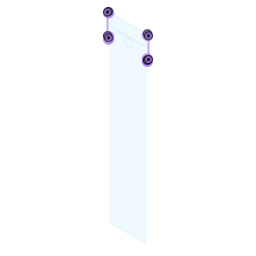
final project_ duck lamp (Autodesk Fusion 360 design; units mm, degrees)
Autodesk Fusion 360 part; units mm, degrees
note: some values were not read from the file. Set by a fixed rule: which sketch regions a step uses.
sketch "Sketch1" plane through (0, 0, 0) normal (0, 1, 0) x (1, 0, 0) in component "back piece"
  line L0 (0, 0) -> (80, 0)
  line L1 (80, 0) -> (80, -347.5)
  line L2 (80, -400) -> (0, -400)
  line L3 (0, -347.5) -> (0, 0)
  line L4 (9, 0) -> (11, 0)
  line L5 (75, -375) -> (5, -375)
  line L6 (5, -375) -> (5, -372)
  line L7 (5, -372) -> (75, -372)
  line L8 (75, -372) -> (75, -375)
  circle A0 centre (40, -363.2398) radius 8.7602
  line L9 (44.9524, -352.3526) -> (35, -352.3526)
  line L10 (35, -352.3526) -> (35, 0)
  line L11 (35, 0) -> (44.9524, 0)
  line L12 (44.9524, 0) -> (44.9524, -352.3526)
  line L13 (0, 0) -> (3, 0)
  line L14 (3, 0) -> (3, -3)
  line L15 (3, -3) -> (0, -3)
  line L16 (80, 0) -> (77, 0)
  line L17 (77, 0) -> (77, -3)
  line L18 (77, -3) -> (80, -3)
  line L19 (80, -3) -> (80, 0)
  line L20 (85, -352.5) -> (85, -397.5)
  line L21 (82.5, -400) -> (-2.5, -400)
  line L22 (-5, -397.5) -> (-5, -352.5)
  line L23 (-2.4999, -350) -> (-2.5, -350)
  line L24 (82.4999, -350) -> (82.5001, -350)
  arc A1 (-2.5, -350) -> (0, -347.5) centre (-2.5, -347.5) ccw
  arc A2 (80, -347.5) -> (82.4999, -350) centre (82.5, -347.5) ccw
  arc A3 (-2.4999, -350) -> (-5, -352.5) centre (-2.5, -352.5) ccw
  arc A4 (85, -352.5) -> (82.5001, -350) centre (82.5, -352.5) ccw
  arc A5 (-5, -397.5) -> (-2.5, -400) centre (-2.5, -397.5) ccw
  arc A6 (82.5, -400) -> (85, -397.5) centre (82.5, -397.5) ccw
  dimension "d5" = 400
  dimension "d6" = 80
  dimension "d98" = 3
  dimension "d99" = 70
  dimension "d115" = 3
  dimension "d116" = 3
  dimension "d117" = 3
  dimension "d118" = 3
  dimension "d121" = 2.5
  dimension "d122" = 2.5
  dimension "d123" = 2.5
  dimension "d124" = 2.5
  dimension "d125" = 2.5
  dimension "d126" = 2.5
  constraint horizontal L0
  constraint vertical L1
  constraint horizontal L2
  constraint vertical L3
  constraint coincident L0.start L3.end
  constraint horizontal L4
  constraint coincident L0 L4.start
  constraint horizontal L5
  constraint vertical L6
  constraint horizontal L7
  constraint vertical L8
  constraint tangent L7 A0
  constraint horizontal L9
  constraint vertical L10
  constraint horizontal L11
  constraint vertical L12
  constraint coincident L0 L10.end
  constraint horizontal L13
  constraint vertical L14
  constraint horizontal L15
  constraint horizontal L16
  constraint vertical L17
  constraint horizontal L18
  constraint vertical L19
  constraint vertical L20
  constraint horizontal L21
  constraint vertical L22
  constraint tangent L3 A1
  constraint tangent L1 A2
  constraint tangent L22 A3
  constraint tangent L20 A4
  constraint tangent L24 A4
  constraint tangent L22 A5
  constraint tangent L21 A5
  constraint tangent L21 A6
  constraint tangent L20 A6
  measures "d5" distance of L0 L2
  measures "d6" distance of L1 L3
  measures "d98" distance of L5 L7
  measures "d99" distance of L6 L8
  measures "d115" distance of L3 L14
  measures "d116" distance of L0 L15
  measures "d117" distance of L0 L18
  measures "d118" distance of L1 L17
  measures "d121" radius of A1
  measures "d122" radius of A2
  measures "d123" radius of A3
  measures "d124" radius of A4
  measures "d125" radius of A5
  measures "d126" radius of A6
sketch "Sketch1 (2)" plane through (0, 0, 0) normal (0, 0, 1) x (1, 0, 0) in component "bottom base"
  line L0 (0, 0) -> (200, 0)
  line L1 (200, 0) -> (200, 106)
  line L2 (200, 106) -> (0, 106)
  line L3 (0, 106) -> (0, 0)
  circle A0 centre (158.3517, 50) radius 35.4262
  circle A1 centre (78.412, 50) radius 35.3232
  line L4 (28.714, 90) -> (25.714, 90)
  line L5 (25.714, 90) -> (25.714, 16)
  line L6 (25.714, 16) -> (28.714, 16)
  line L7 (28.714, 16) -> (28.714, 90)
  dimension "d8" = 200
  dimension "d11" = 106
  dimension "d110" = 3
  dimension "d111" = 74
  dimension "d112" = 16
  dimension "d113" = 10
  dimension "d114" = 25.714
  constraint horizontal L0
  constraint vertical L1
  constraint horizontal L2
  constraint vertical L3
  constraint coincident L0.start L3.end
  constraint horizontal L4
  constraint vertical L5
  constraint horizontal L6
  constraint vertical L7
  measures "d8" distance of L1 L3
  measures "d11" distance of L0 L2
  measures "d110" distance of L5 L7
  measures "d111" distance of L4 L6
  measures "d112" distance of L2 L4
  measures "d114" distance of L3 L5
sketch "Sketch1 (3)" plane through (0, 0, 0) normal (0, 0, 1) x (1, 0, 0) in component "top base"
  line L0 (0, 0) -> (200, 0)
  line L1 (200, 0) -> (200, 100)
  line L2 (200, 100) -> (0, 100)
  line L3 (0, 100) -> (0, 0)
  line L4 (34, 100) -> (34, 0) construction
  line L5 (4, 100) -> (4, 0) construction
  line L6 (-26, 100) -> (-26, 0) construction
  line L7 (-56, 100) -> (-56, 0) construction
  line L8 (0, 50) -> (200, 50) construction
  line L9 (0, 90) -> (200, 90) construction
  line L10 (0, 10) -> (200, 10) construction
  line L11 (159.8571, 90) -> (182.7143, 90)
  line L12 (182.7143, 90) -> (182.7143, 87)
  line L13 (182.7143, 87) -> (159.8571, 87)
  line L14 (159.8571, 87) -> (159.8571, 90)
  line L15 (205.5714, 90) -> (228.4286, 90)
  line L16 (228.4286, 90) -> (228.4286, 87)
  line L17 (228.4286, 87) -> (205.5714, 87)
  line L18 (205.5714, 87) -> (205.5714, 90)
  line L19 (251.2857, 90) -> (274.1429, 90)
  line L20 (274.1429, 90) -> (274.1429, 87)
  line L21 (274.1429, 87) -> (251.2857, 87)
  line L22 (251.2857, 87) -> (251.2857, 90)
  line L23 (159.8571, 10) -> (182.7143, 10)
  line L24 (182.7143, 10) -> (182.7143, 13)
  line L25 (182.7143, 13) -> (159.8571, 13)
  line L26 (159.8571, 13) -> (159.8571, 10)
  line L27 (205.5714, 10) -> (228.4286, 10)
  line L28 (228.4286, 10) -> (228.4286, 13)
  line L29 (228.4286, 13) -> (205.5714, 13)
  line L30 (205.5714, 13) -> (205.5714, 10)
  line L31 (251.2857, 10) -> (274.1429, 10)
  line L32 (274.1429, 10) -> (274.1429, 13)
  line L33 (274.1429, 13) -> (251.2857, 13)
  line L34 (251.2857, 13) -> (251.2857, 10)
  line L35 (174.1429, 42) -> (177.1429, 42)
  line L36 (177.1429, 42) -> (177.1429, 26)
  line L37 (177.1429, 26) -> (174.1429, 26)
  line L38 (174.1429, 26) -> (174.1429, 42)
  line L39 (37, 100) -> (37, 0) construction
  line L40 (197, 100) -> (197, 0) construction
  line L41 (56.8571, 74) -> (59.8571, 74)
  line L42 (59.8571, 74) -> (59.8571, 58)
  line L43 (59.8571, 58) -> (56.8571, 58)
  line L44 (56.8571, 58) -> (56.8571, 74)
  line L45 (56.8571, 42) -> (59.8571, 42)
  line L46 (59.8571, 42) -> (59.8571, 26)
  line L47 (59.8571, 26) -> (56.8571, 26)
  line L48 (56.8571, 26) -> (56.8571, 42)
  line L49 (174.1429, 58) -> (177.1429, 58)
  line L50 (177.1429, 58) -> (177.1429, 74)
  line L51 (177.1429, 74) -> (174.1429, 74)
  line L52 (174.1429, 74) -> (174.1429, 58)
  line L53 (34, 90) -> (37, 90)
  line L54 (37, 90) -> (37, 10)
  line L55 (37, 10) -> (34, 10)
  line L56 (34, 10) -> (34, 90)
  dimension "d18" = 200
  dimension "d19" = 100
  dimension "d20" = 166
  dimension "d21" = 30
  dimension "d22" = 30
  dimension "d23" = 30
  dimension "d30" = 44
  dimension "d31" = 10
  dimension "d32" = 10
  dimension "d34" = 3
  dimension "d35" = 3
  dimension "d36" = 3
  dimension "d40" = 3
  dimension "d41" = 3
  dimension "d42" = 3
  dimension "d46" = 22.8571
  dimension "d47" = 22.8571
  dimension "d48" = 22.8571
  dimension "d49" = 22.8571
  dimension "d50" = 22.8571
  dimension "d51" = 3
  dimension "d52" = 3
  dimension "d54" = 22.8571
  dimension "d55" = 22.8571
  dimension "d56" = 22.8571
  dimension "d57" = 22.8571
  dimension "d58" = 22.8571
  dimension "d59" = 22.8571
  dimension "d61" = 22.8571
  dimension "d80" = 16
  dimension "d81" = 19.8571
  dimension "d83" = 16
  dimension "d84" = 16
  dimension "d85" = 16
  dimension "d86" = 16
  dimension "d87" = 16
  dimension "d88" = 16
  dimension "d89" = 16
  dimension "d90" = 16
  dimension "d91" = 16
  dimension "d92" = 3
  dimension "d93" = 19.8571
  dimension "d94" = 19.8571
  dimension "d95" = 19.8571
  dimension "d96" = 3
  dimension "d97" = 3
  dimension "d104" = 80
  dimension "d105" = 3
  dimension "d106" = 80
  dimension "d107" = 160
  dimension "d108" = 120.2857
  dimension "d109" = 80
  constraint horizontal L0
  constraint vertical L1
  constraint horizontal L2
  constraint vertical L3
  constraint coincident L0.start L3.end
  constraint coincident L2 L4.start
  constraint perpendicular L2 L4
  constraint coincident L2 L5.start
  constraint coincident L0 L5.end
  constraint perpendicular L0 L5
  constraint coincident L2 L6.start
  constraint coincident L0 L6.end
  constraint perpendicular L0 L6
  constraint coincident L2 L7.start
  constraint coincident L0 L7.end
  constraint perpendicular L0 L7
  constraint midpoint L3 L8.start
  constraint midpoint L1 L8.end
  constraint coincident L3 L9.start
  constraint coincident L1 L9.end
  constraint perpendicular L1 L9
  constraint coincident L3 L10.start
  constraint coincident L1 L10.end
  constraint perpendicular L1 L10
  constraint horizontal L11
  constraint vertical L12
  constraint horizontal L13
  constraint vertical L14
  constraint coincident L9 L11.start
  constraint horizontal L15
  constraint vertical L16
  constraint horizontal L17
  constraint vertical L18
  constraint coincident L9 L15.start
  constraint horizontal L19
  constraint vertical L20
  constraint horizontal L21
  constraint vertical L22
  constraint coincident L9 L19.start
  constraint horizontal L23
  constraint vertical L24
  constraint horizontal L25
  constraint vertical L26
  constraint coincident L10 L23.start
  constraint horizontal L27
  constraint vertical L28
  constraint horizontal L29
  constraint vertical L30
  constraint coincident L10 L27.start
  constraint horizontal L31
  constraint vertical L32
  constraint horizontal L33
  constraint vertical L34
  constraint coincident L10 L31.start
  constraint horizontal L35
  constraint vertical L36
  constraint horizontal L37
  constraint vertical L38
  constraint coincident L2 L39.start
  constraint coincident L0 L39.end
  constraint perpendicular L0 L39
  constraint coincident L2 L40.start
  constraint coincident L0 L40.end
  constraint perpendicular L0 L40
  constraint horizontal L41
  constraint vertical L42
  constraint horizontal L43
  constraint vertical L44
  constraint horizontal L45
  constraint vertical L46
  constraint horizontal L47
  constraint vertical L48
  constraint horizontal L49
  constraint vertical L50
  constraint horizontal L51
  constraint vertical L52
  constraint horizontal L53
  constraint vertical L54
  constraint horizontal L55
  constraint vertical L56
  constraint coincident L39 L54.end
  constraint coincident L10 L54.end
  constraint coincident L4 L53.start
  constraint coincident L9 L53.start
  measures "d18" distance of L1 L3
  measures "d19" distance of L0 L2
  measures "d20" distance of L1 L4
  measures "d21" distance of L4 L5
  measures "d22" distance of L5 L6
  measures "d23" distance of L6 L7
  measures "d31" distance of L2 L9
  measures "d32" distance of L0 L10
  measures "d34" distance of L9 L13
  measures "d35" distance of L9 L17
  measures "d36" distance of L9 L21
  measures "d40" distance of L23 L25
  measures "d41" distance of L10 L29
  measures "d42" distance of L10 L33
  measures "d46" distance of L12 L14
  measures "d47" distance of L16 L18
  measures "d48" distance of L20 L22
  measures "d49" distance of L12 L18
  measures "d50" distance of L16 L22
  measures "d51" distance of L1 L40
  measures "d52" distance of L4 L39
  measures "d55" distance of L24 L26
  measures "d56" distance of L28 L30
  measures "d57" distance of L24 L30
  measures "d58" distance of L28 L34
  measures "d59" distance of L32 L34
  measures "d80" distance of L9 L41
  measures "d81" distance of L39 L44
  measures "d83" distance of L41 L43
  measures "d84" distance of L43 L45
  measures "d85" distance of L45 L47
  measures "d86" distance of L23 L47
  measures "d87" distance of L10 L37
  measures "d88" distance of L35 L37
  measures "d89" distance of L35 L49
  measures "d90" distance of L49 L51
  measures "d91" distance of L9 L51
  measures "d92" distance of L50 L52
  measures "d93" distance of L40 L50
  measures "d94" distance of L36 L40
  measures "d95" distance of L39 L48
  measures "d96" distance of L46 L48
  measures "d97" distance of L42 L44
  measures "d104" distance of L53 L55
  measures "d105" distance of L36 L38
  measures "d106" distance of L9 L10
  measures "d107" distance of L40 L54
  measures "d108" distance of L36 L48
  measures "d109" distance of L15 L27
sketch "Sketch1 (4)" plane through (0, 0, 0) normal (0, 0, 1) x (1, 0, 0) in component "top"
  line L0 (0, 0) -> (70, 0)
  line L1 (70, 0) -> (70, 100)
  line L2 (70, 100) -> (0, 100)
  line L3 (0, 100) -> (0, 0)
  dimension "d25" = 100
  dimension "d26" = 70
  constraint horizontal L0
  constraint vertical L1
  constraint horizontal L2
  constraint vertical L3
  constraint coincident L0.start L3.end
  measures "d25" distance of L0 L2
  measures "d26" distance of L1 L3
sketch "Sketch2" plane through (40, 0, 373.5) normal (0, 1, 0) x (1, 0, 0) in component "back piece"
sketch "Sketch2 (2)" plane through (0, 0, 0) normal (0, 0, 1) x (1, 0, 0) in component "bottom base"
sketch "Sketch2 (3)" plane through (0, 0, 0) normal (0, 0, 1) x (1, 0, 0) in component "top base"
sketch "Sketch2 (4)" plane through (0, 0, 0) normal (0, 0, 1) x (1, 0, 0)
sketch "Sketch3" plane through (0, 0, 0) normal (0, 0, 1) x (1, 0, 0)
sketch "Sketch2 (5)" plane through (0, 0, 0) normal (0, 0, 1) x (1, 0, 0) in component "top"
sketch "Sketch3 (2)" plane through (40, 0, 200) normal (0, 1, 0) x (1, 0, 0) in component "back piece"
sketch "Sketch3 (3)" plane through (0, 0, 0) normal (0, 0, 1) x (1, 0, 0) in component "bottom base"
extrude "Extrude1" add sketch "Sketch1" along normal blind 3 contours L0 L1 L2 L3 L4 L9 L10 L12 L14 L15 L17 L18 L20 L21 L22 A1 A2 A3 A4 A5 A6 | L0 L9 L10 L11 L12 in component "back piece"
sketch "Sketch4" plane through (0, 0, 0) normal (0, -1, 0) x (1, 0, 0) in component "back piece"
  circle A0 centre (40, 363.2398) radius 8.7602
  line L0 (40, 372) -> (5, 372)
  line L1 (5, 372) -> (5, 375)
  line L2 (5, 375) -> (75, 375)
  line L3 (75, 375) -> (75, 372)
  line L4 (75, 372) -> (40, 372)
  line L5 (3, 3) -> (3, 0)
  line L6 (3, 0) -> (77, 0)
  line L7 (77, 0) -> (77, 3)
  line L8 (77, 3) -> (80, 3)
  line L9 (80, 3) -> (80, 347.5)
  line L10 (82.5, 400) -> (-2.5, 400)
  line L11 (0, 347.5) -> (0, 3)
  line L12 (0, 3) -> (3, 3)
  arc A1 (82.4999, 350) -> (80, 347.5) centre (82.5, 347.5) ccw
  line L13 (82.4999, 350) -> (82.5001, 350)
  arc A2 (82.5001, 350) -> (85, 352.5) centre (82.5, 352.5) ccw
  line L14 (85, 352.5) -> (85, 397.5)
  arc A3 (85, 397.5) -> (82.5, 400) centre (82.5, 397.5) ccw
  arc A4 (-2.5, 400) -> (-5, 397.5) centre (-2.5, 397.5) ccw
  line L15 (-5, 397.5) -> (-5, 352.5)
  arc A5 (-5, 352.5) -> (-2.4999, 350) centre (-2.5, 352.5) ccw
  arc A6 (0, 347.5) -> (-2.4999, 350) centre (-2.5, 347.5) ccw
component "back piece" placed x (1, 0, 0) y (0, 1, 0) z (0, 0, 1) at (0, 0, 0)
component "bottom base" placed x (1, 0, 0) y (0, 1, 0) z (0, 0, 1) at (0, 0, 0)
component "top base" placed x (1, 0, 0) y (0, 1, 0) z (0, 0, 1) at (0, 0, 0)
component "top" placed x (1, 0, 0) y (0, 1, 0) z (0, 0, 1) at (0, 0, 0)
equation "length_box = 160 mm"
equation "width_box = 80 mm"
equation "thickness = 3 mm"
equation "height = 400 mm"
equation "d5 = height"
equation "d6 = width_box"
equation "d8 = length_base"
equation "length_base = 200 mm"
equation "width_base = 100 mm"
equation "d11 = width_base + 6 mm"
equation "lfinger = 3" comment "number of fingers for length"
equation "wfinger = 2" comment "number of fingers for width"
equation "d18 = length_base"
equation "d19 = width_base"
equation "d20 = length_box + ( 2 * thickness )"
equation "d21 = buffer"
equation "d22 = buffer"
equation "d23 = buffer"
equation "length_top = 70 mm"
equation "d25 = length_top + 30 mm"
equation "d26 = length_top"
equation "width_back = 94 mm"
equation "buffer = 30 mm"
equation "d31 = ( width_base - width_box ) / 2"
equation "d32 = d31"
equation "d34 = thickness"
equation "d35 = thickness"
equation "d36 = thickness"
equation "d40 = thickness"
equation "d41 = thickness"
equation "d42 = thickness"
equation "d46 = length_box / ( 2 * lfinger + 1 )"
equation "d47 = d46"
equation "d48 = d47"
equation "d49 = d46"
equation "d50 = d47"
equation "d51 = thickness"
equation "d52 = thickness"
equation "d53 = d46"
equation "d55 = d53"
equation "d56 = d55"
equation "d57 = d55"
equation "d58 = d56"
equation "d59 = d58"
equation "d62 = width_box / ( 2 * wfinger ) + 1 mm"
equation "d63 = d62"
equation "d66 = width_box / ( 2 * wfinger ) + 1 mm"
equation "d68 = d62"
equation "d70 = d66"
equation "d71 = d70"
equation "d75 = d59"
equation "d78 = d46"
equation "d80 = width_box / ( 2 * wfinger + 1 )"
equation "d81 = d46 - thickness"
equation "d83 = d80"
equation "d84 = d83"
equation "d85 = d84"
equation "d87 = d85"
equation "d88 = d87"
equation "d89 = d88"
equation "d90 = d89"
equation "d92 = thickness"
equation "d93 = d81"
equation "d94 = d95"
equation "d95 = d81"
equation "d96 = thickness"
equation "d97 = thickness"
equation "d98 = thickness"
equation "d99 = width_top"
equation "width_top = 70 mm"
equation "d105 = thickness"
equation "d110 = thickness"
equation "d111 = 80 mm - 6 mm"
equation "d112 = 10 mm + 6 mm"
equation "d115 = thickness"
equation "d116 = thickness"
equation "d117 = thickness"
equation "d118 = thickness"
